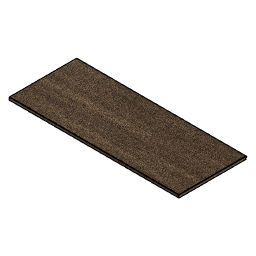
Leaf_End (Autodesk Fusion 360 design; units mm, degrees)
Autodesk Fusion 360 part; units mm, degrees
sketch "Sketch1" plane through (0, 0, 0) normal (0, 0, 1) x (1, 0, 0)
  line L0 (-520.7, 208.28) -> (520.7, 208.28)
  line L1 (520.7, 208.28) -> (520.7, -208.28)
  line L2 (520.7, -208.28) -> (-520.7, -208.28)
  line L3 (-520.7, -208.28) -> (-520.7, 208.28)
  line L4 (-520.7, 208.28) -> (520.7, -208.28) construction
  line L5 (520.7, 208.28) -> (-520.7, -208.28) construction
  dimension "d1" = 416.56
  dimension "d2" = 1041.4
  constraint horizontal L0
  constraint perpendicular L0 L1
  constraint parallel L0 L2
  constraint parallel L1 L3
  constraint coincident L4 origin
  constraint coincident L5 origin
  measures "d1" distance of L0.end L1.end
  measures "d2" distance of L0.start L0.end
extrude "Extrude1" add sketch "Sketch1" along normal blind 19.05
sketch "Sketch3" plane through (520.7, 0, 0) normal (1, 0, 0) x (0, 1, 0)
  line L0 (-208.28, 0) -> (208.28, 0)
  line L1 (208.28, 0) -> (208.28, 19.05)
  line L2 (208.28, 19.05) -> (-208.28, 19.05)
  line L3 (-208.28, 19.05) -> (-208.28, 0)
  line L4 (204.47, 0) -> (204.47, 3.175)
  line L5 (204.47, 15.875) -> (204.47, 19.05)
  line L6 (204.47, 3.175) -> (200.66, 4.1959)
  line L7 (200.66, 4.1959) -> (200.66, 8.5041)
  line L8 (200.66, 8.5041) -> (204.47, 9.525)
  line L9 (208.28, 10.5459) -> (208.28, 14.8541) construction
  line L10 (208.28, 14.8541) -> (204.47, 15.875)
  line L11 (204.47, 9.525) -> (208.28, 10.5459)
  line L12 (204.47, 0) -> (208.28, 0)
  line L13 (204.47, 19.05) -> (208.28, 19.05)
  line L14 (208.28, 19.05) -> (208.28, 14.8541)
  line L15 (208.28, 0) -> (208.28, 10.5459)
  point P0 (208.28, 0)
  dimension "d25" = 105
  dimension "d27" = 19.05
  dimension "d29" = 6.35
  dimension "d30" = 6.35
  dimension "d31" = 3.81
  dimension "d32" = 3.81
  dimension "d33" = 3.81
  constraint vertical L4
  constraint vertical L5
  constraint equal L6 L10
  constraint parallel L6 L10
  constraint equal L4 L5
  constraint equal L7 L9
  constraint equal L8 L11
  constraint equal L6 L8
  constraint perpendicular L9 L12
  constraint perpendicular L5 L13
  constraint perpendicular L13 L14
  constraint perpendicular L12 L15
  measures "d25" angle of L6 L7
  measures "d27" distance of L4.start L5.end
  measures "d29" distance of L5.start L8.end
  measures "d30" distance of L4.end L8.end
  measures "d31" distance of L7 L8.end
  measures "d32" distance of L9 L8.end
  measures "d33" distance of L4.start P0
extrude "Extrude3" cut sketch "Sketch3" against normal blind 1041.4 contours L0 L1 L4 L6 L7 L8 L11 L12 L15 | L1 L2 L5 L10 L13 L14
chamfer "Chamfer1" distance 1.5875 angle 45 8 edges at (-520.7, -1.905, 19.05) (520.7, -1.905, 19.05) (-520.7, -1.905, 0) (520.7, -1.905, 0) (0, -208.28, 0) (0, -208.28, 19.05) (0, 204.47, 19.05) (0, 204.47, 0)
